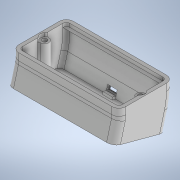
# Autodesk Inventor part: Case
Saved by Autodesk Inventor 2020 (Build 240168000, 168)
## iProperties
Created: 2021-04-19
Part Number: Case
Material: Generic
Document SubType Name: Modeling
Designer: user
Density: 1 g/cm^3
Appearance: Default
Author: user
Autodesk Inventor part; units mm, degrees
ref_plane "YZ Plane" through (0, 0, 0) normal (1, 0, 0) x (0, 1, 0)
ref_plane "XZ Plane" through (0, 0, 0) normal (0, 1, 0) x (-1, 0, 0)
ref_plane "XY Plane" through (0, 0, 0) normal (0, 0, 1) x (1, 0, 0)
sketch "Sketch1" plane through (0, 0, 0) normal (0, 0, 1) x (1, 0, 0)
  line L0 (2.54, 0) -> (81.28, 0)
  line L1 (81.28, 39.37) -> (2.54, 39.37)
  circle A0 centre (1.27, 19.685) radius 1.6
  circle A1 centre (82.55, 19.685) radius 1.6
  arc A2 (2.54, 39.37) -> (0, 36.83) centre (2.54, 36.83) ccw
  arc A3 (83.82, 36.83) -> (81.28, 39.37) centre (81.28, 36.83) ccw
  arc A4 (81.28, 0) -> (83.82, 2.54) centre (81.28, 2.54) ccw
  arc A5 (0, 2.54) -> (2.54, 0) centre (2.54, 2.54) ccw
  arc A6 (-0.8467, 22.0515) -> (-0.8467, 17.3185) centre (1.27, 19.685) ccw
  arc A7 (84.6667, 17.3185) -> (84.6667, 22.0515) centre (82.55, 19.685) ccw
  line L2 (0, 36.83) -> (0, 23.9447)
  line L3 (0, 15.4253) -> (0, 2.54)
  line L4 (83.82, 2.54) -> (83.82, 15.4253)
  line L5 (83.82, 23.9447) -> (83.82, 36.83)
  arc A8 (-0.8467, 22.0515) -> (0, 23.9447) centre (-2.54, 23.9447) ccw
  arc A9 (0, 15.4253) -> (-0.8467, 17.3185) centre (-2.54, 15.4253) ccw
  arc A10 (83.82, 23.9447) -> (84.6667, 22.0515) centre (86.36, 23.9447) ccw
  arc A11 (84.6667, 17.3185) -> (83.82, 15.4253) centre (86.36, 15.4253) ccw
  line L6 (2.54, 39.77) -> (81.28, 39.77)
  arc A12 (84.22, 36.83) -> (81.28, 39.77) centre (81.28, 36.83) ccw
  line L7 (84.22, 36.83) -> (84.22, 23.9447)
  arc A13 (84.22, 23.9447) -> (84.9333, 22.3496) centre (86.36, 23.9447) ccw
  arc A14 (84.9333, 17.0204) -> (84.9333, 22.3496) centre (82.55, 19.685) ccw
  arc A15 (84.9333, 17.0204) -> (84.22, 15.4253) centre (86.36, 15.4253) ccw
  line L8 (84.22, 15.4253) -> (84.22, 2.54)
  arc A16 (81.28, -0.4) -> (84.22, 2.54) centre (81.28, 2.54) ccw
  line L9 (81.28, -0.4) -> (2.54, -0.4)
  arc A17 (-0.4, 2.54) -> (2.54, -0.4) centre (2.54, 2.54) ccw
  line L10 (-0.4, 2.54) -> (-0.4, 15.4253)
  arc A18 (-0.4, 15.4253) -> (-1.1133, 17.0204) centre (-2.54, 15.4253) ccw
  arc A19 (-1.1133, 22.3496) -> (-1.1133, 17.0204) centre (1.27, 19.685) ccw
  arc A20 (-1.1133, 22.3496) -> (-0.4, 23.9447) centre (-2.54, 23.9447) ccw
  line L11 (-0.4, 23.9447) -> (-0.4, 36.83)
  arc A21 (2.54, 39.77) -> (-0.4, 36.83) centre (2.54, 36.83) ccw
  line L12 (-0.4, 23.9447) -> (-0.4, 15.4253)
  line L13 (84.22, 23.9447) -> (84.22, 15.4253)
  line L14 (87.22, 22.5161) -> (87.22, 36.83)
  arc A22 (87.22, 36.83) -> (81.28, 42.77) centre (81.28, 36.83) ccw
  line L15 (81.28, 42.77) -> (2.54, 42.77)
  arc A23 (2.54, 42.77) -> (-3.4, 36.83) centre (2.54, 36.83) ccw
  line L16 (-3.4, 36.83) -> (-3.4, 22.5161)
  line L17 (-3.4, 15.4253) -> (-3.4, 2.54)
  arc A24 (-3.4, 2.54) -> (2.54, -3.4) centre (2.54, 2.54) ccw
  line L18 (2.54, -3.4) -> (81.28, -3.4)
  arc A25 (81.28, -3.4) -> (87.22, 2.54) centre (81.28, 2.54) ccw
  line L19 (87.22, 2.54) -> (87.22, 13.9967)
  line L20 (-3.4, 22.5161) -> (-3.4, 15.4253)
  line L21 (87.22, 22.5161) -> (87.22, 13.9967)
  line L22 (-0.4, 37.27) -> (84.22, 37.27)
  line L23 (-0.4, 2.1) -> (84.22, 2.1)
  circle A26 centre (1.27, 19.685) radius 3.575
  circle A27 centre (82.55, 19.685) radius 3.575
  line L24 (1.27, 23.26) -> (-0.4, 23.9447)
  line L25 (1.27, 16.11) -> (-0.4, 15.4253)
  line L26 (82.55, 16.11) -> (84.22, 15.4253)
  line L27 (82.55, 23.26) -> (84.22, 23.9447)
  point P0 (0, 0)
  point P1 (83.82, 39.37)
  point P2 (83.82, 0)
  point P3 (0, 39.37)
  point P4 (41.91, 39.37)
  point P5 (0, 22.5949)
  point P6 (0, 16.7751)
  point P7 (83.82, 16.7751)
  point P8 (83.82, 22.5949)
  dimension "d0" = 83.82
  dimension "d1" = 39.37
  dimension "d2" = 3.2
  dimension "d3" = 3.2
  dimension "d4" = 81.28
  dimension "d5" = 40.64
  dimension "d6" = 2.54
  dimension "d7" = 6.35
  dimension "d8" = 6.35
  dimension "d9" = 2.54
  dimension "d10" = 0.4
  dimension "d11" = 3
  dimension "d12" = 3
  dimension "d13" = 2.5
  dimension "d14" = 2.5
  dimension "d109" = 46.17
  dimension "d110" = 23.085
  dimension "d111" = 23.085
  constraints: 56 end point, 56 point on circle, 28 centre point, 22 tangent, 16 parallel, 12 point on line, 8 equal radius, 7 perpendicular, 4 coincident, 1 horizontal, 1 midpoint, 1 vertical, 23 other
  measures "d0" distance of point (0, 39.37) point (83.82, 39.37)
  measures "d1" distance of point (83.82, 39.37) point (83.82, 0)
  measures "d2" diameter of A0
  measures "d3" diameter of A1
  measures "d4" distance of A1.centre A0.centre
  measures "d5" horizontal distance of A0.centre point (41.91, 39.37)
  measures "d6" radius of A2
  measures "d7" diameter of A6
  measures "d8" diameter of A7
  measures "d9" radius of A8
  measures "d10" distance between parallel lines of L1 L6
  measures "d11" distance between parallel lines of L6 L15
  measures "d12" distance between parallel lines of L9 L18
  measures "d13" distance between parallel lines of L22 L6
  measures "d14" distance between parallel lines of L9 L23
  measures "d109" distance between parallel lines of L15 L18
  measures "d110" distance from line of L15 A0.centre
  measures "d111" distance from line of L15 A1.centre
extrude "Extrusion1" add sketch "Sketch1" along normal blind 3 contours L21 L19 A25 L18 A24 L17 L20 L16 A23 L15 A22 L14
sketch "Sketch2" plane through (0, 0, 0) normal (0, 0, -1) x (-1, 0, 0)
  line L0 (-81.28, 42.77) -> (-2.54, 42.77)
  line L1 (3.4, 36.83) -> (3.4, 2.54)
  line L2 (-2.54, -3.4) -> (-81.28, -3.4)
  line L3 (-87.22, 2.54) -> (-87.22, 36.83)
  arc A0 (-81.28, 42.77) -> (-87.22, 36.83) centre (-81.28, 36.83) ccw
  arc A1 (-87.22, 2.54) -> (-81.28, -3.4) centre (-81.28, 2.54) ccw
  arc A2 (-2.54, -3.4) -> (3.4, 2.54) centre (-2.54, 2.54) ccw
  arc A3 (3.4, 36.83) -> (-2.54, 42.77) centre (-2.54, 36.83) ccw
  line L4 (-2.54, 39.77) -> (-81.28, 39.77)
  arc A4 (-81.28, 39.77) -> (-84.22, 36.83) centre (-81.28, 36.83) ccw
  line L5 (-84.22, 36.83) -> (-84.22, 2.54)
  arc A5 (-84.22, 2.54) -> (-81.28, -0.4) centre (-81.28, 2.54) ccw
  line L6 (-81.28, -0.4) -> (-2.54, -0.4)
  arc A6 (-2.54, -0.4) -> (0.4, 2.54) centre (-2.54, 2.54) ccw
  line L7 (0.4, 2.54) -> (0.4, 36.83)
  arc A7 (0.4, 36.83) -> (-2.54, 39.77) centre (-2.54, 36.83) ccw
  arc A8 (-84.9333, 22.3496) -> (-84.9333, 17.0204) centre (-82.55, 19.685) ccw projected
  circle A9 centre (-82.55, 19.685) radius 3.575
  arc A10 (1.1133, 17.0204) -> (1.1133, 22.3496) centre (-1.27, 19.685) ccw projected
  circle A11 centre (-1.27, 19.685) radius 3.575
  line L8 (-84.22, 36.83) -> (-84.22, 23.9447) projected
  line L9 (-84.22, 36.77) -> (0.4, 36.77)
  line L10 (0.4, 23.9447) -> (0.4, 36.83) projected
  line L11 (-84.22, 15.4253) -> (-84.22, 2.54) projected
  line L12 (-84.22, 2.6) -> (0.4, 2.6)
  line L13 (0.4, 2.54) -> (0.4, 15.4253) projected
  arc A12 (-84.9333, 22.3496) -> (-84.22, 23.9447) centre (-86.36, 23.9447) ccw projected
  line L14 (-82.55, 23.26) -> (-84.22, 23.9447)
  line L15 (-84.22, 15.4253) -> (-82.55, 16.11)
  arc A13 (0.4, 23.9447) -> (1.1133, 22.3496) centre (2.54, 23.9447) ccw projected
  line L16 (0.4, 23.9447) -> (-1.27, 23.26)
  line L17 (0.4, 15.4253) -> (-1.27, 16.11)
  circle A14 centre (-82.55, 19.685) radius 2
  circle A15 centre (-1.27, 19.685) radius 2
  point P0 (0, 0)
  point P1 (0.4, 2.6)
  point P2 (0.4, 36.77)
  dimension "d17" = 5.94
  dimension "d18" = 3
  dimension "d19" = 3
  dimension "d20" = 3
  dimension "d21" = 4
  dimension "d22" = 4
  constraints: 28 end point, 20 point on circle, 12 centre point, 8 tangent, 5 parallel, 4 coincident, 4 perpendicular, 4 point on line, 3 equal radius, 1 horizontal, 7 other
  measures "d17" radius of A0
  measures "d18" distance between parallel lines of L0 L4
  measures "d19" distance between parallel lines of L9 L4
  measures "d20" distance between parallel lines of L6 L12
  measures "d21" diameter of A14
  measures "d22" diameter of A15
extrude "Extrusion2" add sketch "Sketch2" along normal blind 3 contours L0 A3 L1 A2 L2 A1 L3 A0 | A7 L7 L9 L5 A4 L4 | A13 A11 L7 | L7 A11 L16 | L14 A9 L5 | L5 A9 A12 | A11 A10 L7 A15 | L7 A15 A11 | A9 L5 A14 | L5 A14 A9 A8 | A11 L7 L17 | A9 L15 L5 | L7 A6 L6 A5 L5 L12
sketch "Sketch3" plane through (0, 0, -3) normal (0, 0, -1) x (-1, 0, 0)
  line L0 (-2.54, -3.4) -> (-81.28, -3.4)
  line L1 (-87.22, 2.54) -> (-87.22, 36.83)
  line L2 (-81.28, 42.77) -> (-2.54, 42.77)
  line L3 (3.4, 36.83) -> (3.4, 2.54)
  arc A0 (-2.54, -3.4) -> (3.4, 2.54) centre (-2.54, 2.54) ccw
  arc A1 (3.4, 36.83) -> (-2.54, 42.77) centre (-2.54, 36.83) ccw
  arc A2 (-81.28, 42.77) -> (-87.22, 36.83) centre (-81.28, 36.83) ccw
  arc A3 (-87.22, 2.54) -> (-81.28, -3.4) centre (-81.28, 2.54) ccw
  line L4 (-81.28, -0.4) -> (-2.54, -0.4)
  arc A4 (-2.54, -0.4) -> (0.4, 2.54) centre (-2.54, 2.54) ccw
  line L5 (0.4, 2.54) -> (0.4, 36.83)
  arc A5 (0.4, 36.83) -> (-2.54, 39.77) centre (-2.54, 36.83) ccw
  line L6 (-2.54, 39.77) -> (-81.28, 39.77)
  arc A6 (-81.28, 39.77) -> (-84.22, 36.83) centre (-81.28, 36.83) ccw
  line L7 (-84.22, 36.83) -> (-84.22, 2.54)
  arc A7 (-84.22, 2.54) -> (-81.28, -0.4) centre (-81.28, 2.54) ccw
  line L8 (-7.7403, -13.4) -> (-77.0436, -13.4)
  point P0 (0, 0)
  dimension "d28" = 5.94
  dimension "d29" = 3
  dimension "d30" = 10
  constraints: 18 end point, 16 point on circle, 8 centre point, 8 tangent, 4 parallel, 3 equal radius, 2 horizontal, 2 perpendicular, 7 other
  measures "d28" radius of A0
  measures "d29" distance between parallel lines of L0 L4
  measures "d30" distance between parallel lines of L0 L8
revolve "Revolution1" add sketch "Sketch3" angle 15 about axis through (7.7403, -13.4, -3) along (-1, 0, 0)
chamfer "Chamfer2" distance 3 angle 45 2 edges at (41.91, 36.77, -3) (41.91, 2.6, -3)
sketch "Sketch4" plane through (81.28, -3.7407, -5.5882) normal (0, -0.258819, -0.9659258) x (-1, 0, 0)
  line L0 (0, 46.17) -> (78.74, 46.17)
  line L1 (84.68, 40.23) -> (84.68, 5.94)
  line L2 (78.74, 0) -> (0, 0)
  line L3 (-5.94, 5.94) -> (-5.94, 40.23)
  line L4 (84.68, 5.94) -> (84.68, 40.23) projected
  line L5 (0, 0) -> (78.74, 0) projected
  arc A0 (0, 46.17) -> (-5.94, 40.23) centre (0, 40.23) ccw
  arc A1 (-5.94, 5.94) -> (0, 0) centre (0, 5.94) ccw
  arc A2 (78.74, 0) -> (84.68, 5.94) centre (78.74, 5.94) ccw
  arc A3 (84.68, 40.23) -> (78.74, 46.17) centre (78.74, 40.23) ccw
  line L6 (78.74, 43.17) -> (0, 43.17)
  arc A4 (0, 43.17) -> (-2.94, 40.23) centre (0, 40.23) ccw
  line L7 (-2.94, 40.23) -> (-2.94, 5.94)
  arc A5 (-2.94, 5.94) -> (0, 3) centre (0, 5.94) ccw
  line L8 (0, 3) -> (78.74, 3)
  arc A6 (78.74, 3) -> (81.68, 5.94) centre (78.74, 5.94) ccw
  line L9 (81.68, 5.94) -> (81.68, 40.23)
  arc A7 (81.68, 40.23) -> (78.74, 43.17) centre (78.74, 40.23) ccw
  point P0 (81.28, 2.1669)
  dimension "d35" = 0
  dimension "d36" = 0
  dimension "d37" = 5.94
  dimension "d38" = 3
  constraints: 16 end point, 16 point on circle, 8 centre point, 8 tangent, 4 parallel, 3 equal radius, 2 perpendicular, 1 horizontal, 7 other
  measures "d35" distance between parallel lines of L1 L4
  measures "d36" distance between parallel lines of L5 L2
  measures "d37" radius of A0
  measures "d38" distance between parallel lines of L0 L6
extrude "Extrusion3" add sketch "Sketch4" along normal blind 12
sketch "Sketch5" plane through (81.28, -6.8466, -17.1793) normal (0, -0.258819, -0.9659258) x (-1, 0, 0)
  line L0 (78.74, 46.17) -> (0, 46.17)
  line L1 (-5.94, 40.23) -> (-5.94, 5.94)
  line L2 (0, 0) -> (78.74, 0)
  line L3 (84.68, 5.94) -> (84.68, 40.23)
  line L4 (-5.94, 40.23) -> (-5.94, 5.94) projected
  line L5 (0, 0) -> (78.74, 0) projected
  arc A0 (78.74, 0) -> (84.68, 5.94) centre (78.74, 5.94) ccw
  arc A1 (-5.94, 5.94) -> (0, 0) centre (0, 5.94) ccw
  arc A2 (0, 46.17) -> (-5.94, 40.23) centre (0, 40.23) ccw
  arc A3 (84.68, 40.23) -> (78.74, 46.17) centre (78.74, 40.23) ccw
  point P0 (81.28, 2.1669)
  dimension "d41" = 0
  dimension "d42" = 0
  dimension "d43" = 5.94
  constraints: 8 end point, 8 point on circle, 8 tangent, 4 centre point, 3 equal radius, 2 parallel, 1 horizontal, 1 perpendicular
  measures "d41" distance between parallel lines of L4 L1
  measures "d42" distance between parallel lines of L5 L2
  measures "d43" radius of A0
extrude "Extrusion4" add sketch "Sketch5" along normal blind 4
sketch "Sketch6" plane through (81.28, -7.8818, -21.043) normal (0, -0.258819, -0.9659258) x (-1, 0, 0)
  circle A0 centre (75.68, 9) radius 6.25
  circle A1 centre (75.68, 37.17) radius 6.25
  circle A2 centre (3.06, 9) radius 6.25
  circle A3 centre (3.06, 37.17) radius 6.25
  line L0 (84.68, 5.94) -> (84.68, 40.23) projected
  line L1 (0, 0) -> (78.74, 0) projected
  line L2 (78.74, 46.17) -> (0, 46.17) projected
  line L3 (-5.94, 40.23) -> (-5.94, 5.94) projected
  point P0 (81.28, 2.1669)
  dimension "d46" = 12.5
  dimension "d47" = 12.5
  dimension "d48" = 12.5
  dimension "d49" = 12.5
  dimension "d50" = 9
  dimension "d51" = 9
  dimension "d52" = 9
  dimension "d53" = 9
  dimension "d54" = 9
  dimension "d55" = 9
  dimension "d56" = 9
  dimension "d57" = 9
  constraints: 4 centre point
  measures "d46" diameter of A0
  measures "d47" diameter of A1
  measures "d48" diameter of A2
  measures "d49" diameter of A3
  measures "d50" distance from line of L0 A0.centre
  measures "d51" distance from line of L1 A0.centre
  measures "d52" distance from line of L0 A1.centre
  measures "d53" distance from line of L2 A1.centre
  measures "d54" distance from line of A2.centre L1
  measures "d55" distance from line of L3 A2.centre
  measures "d56" distance from line of L3 A3.centre
  measures "d57" distance from line of L2 A3.centre
extrude "Extrusion5" cut sketch "Sketch6" against normal blind 3
sketch "Sketch8" plane through (81.28, -6.8466, -17.1793) normal (0, 0.258819, 0.9659258) x (1, 0, 0)
  line L0 (-48.47, 10.07) -> (-30.27, 10.07)
  line L1 (-30.27, 10.07) -> (-30.27, 43.17)
  line L2 (-30.27, 43.17) -> (-48.47, 43.17)
  line L3 (-48.47, 43.17) -> (-48.47, 10.07)
  line L4 (0, 43.17) -> (-78.74, 43.17) projected
  line L5 (-43.47, 7.07) -> (-35.27, 7.07)
  line L6 (-35.27, 7.07) -> (-35.27, 13.07)
  line L7 (-35.27, 13.07) -> (-43.47, 13.07)
  line L8 (-43.47, 13.07) -> (-43.47, 7.07)
  line L9 (-43.47, 40.17) -> (-35.27, 40.17)
  line L10 (-35.27, 40.17) -> (-35.27, 43.17)
  line L11 (-35.27, 43.17) -> (-43.47, 43.17)
  line L12 (-43.47, 43.17) -> (-43.47, 40.17)
  line L13 (-81.68, 40.23) -> (-81.68, 5.94) projected
  point P0 (-81.28, 2.1669)
  point P1 (0, 46.17)
  dimension "d70" = 18.2
  dimension "d71" = 33.1
  dimension "d73" = 0
  dimension "d74" = 5
  dimension "d75" = 5
  dimension "d76" = 3
  dimension "d77" = 3
  dimension "d78" = 3
  dimension "d79" = 0
  dimension "d95" = 33.21
  dimension "d96" = 5
  dimension "d97" = 5
  constraints: 24 end point, 6 parallel, 3 horizontal, 3 perpendicular
  measures "d70" distance of L2.end L1.end
  measures "d71" distance of L1.end L0.end
  measures "d73" distance between parallel lines of L2 L4
  measures "d74" distance between parallel lines of L8 L3
  measures "d75" distance between parallel lines of L1 L6
  measures "d76" distance between parallel lines of L0 L5
  measures "d77" distance between parallel lines of L7 L0
  measures "d78" distance of L11.end L9.start
  measures "d79" distance between parallel lines of L4 L11
  measures "d95" distance between parallel lines of L3 L13
  measures "d96" distance between parallel lines of L12 L3
  measures "d97" distance between parallel lines of L1 L10
extrude "Extrusion6" add sketch "Sketch8" along normal blind 2 contours L8 L7 L6 L0 | L0 L6 L5 L8 | L2 L10 L9 L12
sketch "Sketch9" plane through (81.28, -6.3289, -15.2474) normal (0, 0.258819, 0.9659258) x (1, 0, 0)
  line L0 (-35.27, 7.07) -> (-43.47, 7.07) projected
  line L1 (-35.27, 13.07) -> (-35.27, 7.07) projected
  line L2 (-43.47, 7.07) -> (-35.27, 7.07)
  line L3 (-35.27, 7.07) -> (-35.27, 10.07)
  line L4 (-35.27, 10.07) -> (-43.47, 10.07)
  line L5 (-43.47, 10.07) -> (-43.47, 7.07)
  point P0 (-81.28, 2.1669)
  dimension "d82" = 3
  constraints: 8 end point, 2 parallel, 1 horizontal, 1 midpoint, 1 perpendicular
  measures "d82" distance of L3.end L2.end
extrude "Extrusion7" add sketch "Sketch9" along normal blind 3
chamfer "Chamfer3" distance 0.8 angle 45 1 edges at (41.91, 4.1744, -14.956)
sketch "Sketch10" plane through (2.54, 40.8561, -17.5379) normal (0, 0.9659258, -0.258819) x (1, 0, 0)
  line L0 (43.37, 5.8) -> (35.37, 5.8)
  line L1 (35.37, 5.8) -> (35.37, 9.6)
  line L2 (35.37, 9.6) -> (43.37, 9.6)
  line L3 (43.37, 9.6) -> (43.37, 5.8)
  line L4 (0, 0) -> (0, 16) projected
  line L5 (78.74, 0) -> (78.74, 16) projected
  line L6 (0, 16) -> (78.74, 16) projected
  point P0 (-2.54, -6.366)
  dimension "d88" = 8
  dimension "d89" = 3.8
  dimension "d90" = 78.74
  dimension "d91" = 35.37
  dimension "d92" = 6.4
  constraints: 8 end point, 2 parallel, 1 horizontal, 1 perpendicular
  measures "d88" distance of L1.end L2.end
  measures "d89" distance of L0.end L1.end
  measures "d90" distance between parallel lines of L4 L5
  measures "d91" distance between parallel lines of L3 L5
  measures "d92" distance between parallel lines of L2 L6
extrude "Extrusion8" cut sketch "Sketch10" against normal blind 3
sketch "Sketch13" plane through (0, 0, 0) normal (0, 0, 1) x (1, 0, 0)
  arc A0 (-0.4, 18.5845) -> (-0.4, 20.7855) centre (1.27, 19.685) ccw projected
  circle A1 centre (1.27, 19.685) radius 3.575
  line L0 (1.27, 16.11) -> (-0.4, 15.4253) projected
  line L1 (1.27, 16.11) -> (-0.4, 15.4253)
  arc A2 (-0.4, 15.4253) -> (-1.1133, 17.0204) centre (-2.54, 15.4253) ccw projected
  line L2 (-0.4, 15.4253) -> (-1.1133, 17.0204)
  arc A3 (1.27, 16.11) -> (1.27, 23.26) centre (1.27, 19.685) ccw projected
  line L3 (-0.4, 23.9447) -> (1.27, 23.26) projected
  line L4 (1.27, 23.26) -> (-0.4, 23.9447)
  line L5 (-0.4, 23.9447) -> (-1.1133, 22.3496)
  arc A4 (84.22, 20.7855) -> (84.22, 18.5845) centre (82.55, 19.685) ccw projected
  circle A5 centre (82.55, 19.685) radius 3.575
  line L6 (84.22, 15.4253) -> (82.55, 16.11) projected
  line L7 (82.55, 16.11) -> (84.22, 15.4253)
  arc A6 (84.9333, 17.0204) -> (84.22, 15.4253) centre (86.36, 15.4253) ccw projected
  line L8 (84.22, 15.4253) -> (84.9333, 17.0204)
  line L9 (82.55, 23.26) -> (84.22, 23.9447) projected
  line L10 (84.22, 36.83) -> (84.22, 23.9447) projected
  line L11 (82.55, 23.26) -> (84.22, 23.9447)
  line L12 (84.22, 23.9447) -> (84.9333, 22.3496)
  arc A7 (84.22, 23.9447) -> (84.9333, 22.3496) centre (86.36, 23.9447) ccw projected
  point P0 (0, 0)
  constraints: 16 end point, 3 coincident, 3 collinear, 2 centre point, 2 point on circle
extrude "Extrusion10" add sketch "Sketch13" against normal blind 26.75 contours A1 | A1 L5 L3 | L0 A2 A1 | A5 | A5 L9 A7 | A6 L6 A5
sketch "Sketch14" plane through (0, 0, 0) normal (0, 0, 1) x (1, 0, 0)
  arc A0 (1.27, 16.11) -> (1.27, 23.26) centre (1.27, 19.685) ccw projected
  arc A1 (82.55, 23.26) -> (82.55, 16.11) centre (82.55, 19.685) ccw projected
  point P0 (0, 0)
  constraints: 2 coincident
hole "Hole1" at (1.27, 19.685, 0) at (82.55, 19.685, 0) direction (0, 0, -1) diameter 3.5 depth 4.01 countersink diameter 4 countersink angle 7.15
body "Solid1"
